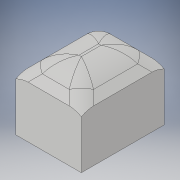
# Autodesk Inventor part: LED2
Saved by Autodesk Inventor 2019 (Build 230136000, 136)
## iProperties
Created: 2018-12-21
Part Number: LED2
Material: Типовые
Document SubType Name: Modeling
Designer: aldanstar
Density: 1 g/cm^3
Appearance: По умолчанию
Author: aldanstar
Autodesk Inventor part; units mm, degrees
ref_plane "YZ Plane" through (0, 0, 0) normal (1, 0, 0) x (0, 1, 0)
ref_plane "XZ Plane" through (0, 0, 0) normal (0, 1, 0) x (-1, 0, 0)
ref_plane "XY Plane" through (0, 0, 0) normal (0, 0, 1) x (1, 0, 0)
sketch "Эскиз1" plane through (0, 0, 0) normal (0, 1, 0) x (-1, 0, 0)
  line L0 (1.9, -2.4) -> (-1.9, -2.4)
  line L1 (-1.9, -2.4) -> (-1.9, 2.4)
  line L2 (-1.9, 2.4) -> (1.9, 2.4)
  line L3 (1.9, 2.4) -> (1.9, -2.4)
  line L4 (0, -2.4) -> (0, 2.4) construction
  line L5 (1.9, 0) -> (-1.9, 0) construction
  line L6 (0, -3.36) -> (0, 3.36) projected
  line L7 (2.66, 0) -> (-2.66, 0) projected
  point P0 (0, 0)
  dimension "d4" = 3.8
  dimension "d5" = 4.8
  constraints: 12 end point, 4 midpoint, 2 parallel, 1 collinear, 1 horizontal, 1 perpendicular, 1 other
  measures "d4" distance of L2.start L3.start
  measures "d5" distance of L3.start L0.start
extrude "Выдавливание1" add sketch "Эскиз1" along normal blind 4
chamfer "Фаска1" distance 1 angle 45 4 edges at (1.9, 4, 0) (0, 4, 2.4) (-1.9, 4, 0) (0, 4, -2.4)
fillet "Сопряжение1" radius 2 4 edges at (0.9, 4, 0) (-0.9, 4, 0) (0, 4, 1.4) (0, 4, -1.4)
fillet "Сопряжение2" radius 1 12 edges at (0, 3.4142, -1.9858) (-1.4858, 3.4142, 0) (1.4858, 3.4142, 0) (0, 3.4142, 1.9858) (-1.6929, 3.2071, -2.1929) (-0.8369, 3.8478, -1.3369) (1.6929, 3.2071, -2.1929) (0.8369, 3.8478, -1.3369) (1.6929, 3.2071, 2.1929) (0.8369, 3.8478, 1.3369) (-1.6929, 3.2071, 2.1929) (-0.8369, 3.8478, 1.3369)
